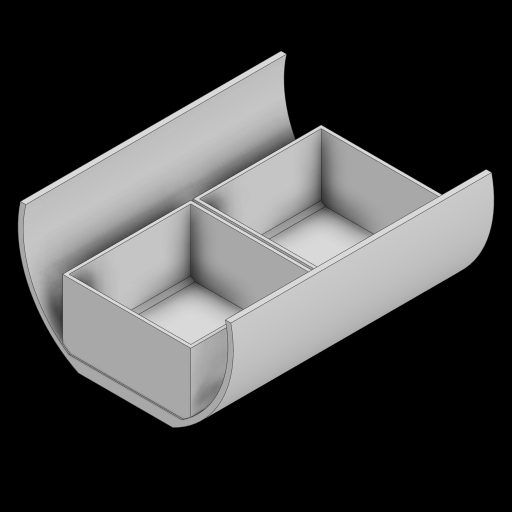
# Autodesk Inventor part: InsertV1
Saved by Autodesk Inventor 2024 (Build 280153000, 153)
## iProperties
Created: 2026-04-20
Part Number: InsertV1
Material: Generic
Document SubType Name: Modeling
Designer: Tanner
Density: 1 g/cm^3
Appearance: Default
Author: Tanner
## iProperties of the stored document InsertV1_3DPrint.ipt
Created: 2026-04-27
Part Number: InsertV1_3DPrint
Material: Generic
Document SubType Name: Modeling
Designer: Tanner
Density: 1 g/cm^3
Appearance: Default
Author: Tanner
Autodesk Inventor part; units mm, degrees
ref_plane "YZ Plane" through (0, 0, 0) normal (1, 0, 0) x (0, 1, 0)
ref_plane "XZ Plane" through (0, 0, 0) normal (0, 1, 0) x (-1, 0, 0)
ref_plane "XY Plane" through (0, 0, 0) normal (0, 0, 1) x (1, 0, 0)
sketch "Sketch1" plane through (0, 0, 0) normal (0, 0, 1) x (1, 0, 0)
  circle A0 centre (0, 0) radius 107.6 construction
  arc A1 (43.4971, -89.6) -> (-43.4971, -89.6) centre (0, 0) ccw construction
  line L0 (43.4971, -89.6) -> (-43.4971, -89.6) construction
  arc A2 (-96.8589, 20.9561) -> (-43.4971, -89.0439) centre (0, 0) ccw
  line L1 (-43.4971, -89.0439) -> (0, -89.0439)
  line L2 (-96.8589, 20.9561) -> (-91.8589, 20.9561)
  arc A3 (-91.8589, 20.9561) -> (-43.4971, -83.5776) centre (0, 0) ccw
  line L3 (-43.4971, -83.5776) -> (0, -83.5776)
  line L4 (0, 99.6) -> (0, -89.6) construction
  arc A4 (43.4971, -89.0439) -> (96.8589, 20.9561) centre (0, 0) ccw
  line L5 (43.4971, -89.0439) -> (0, -89.0439)
  line L6 (96.8589, 20.9561) -> (91.8589, 20.9561)
  arc A5 (43.4971, -83.5776) -> (91.8589, 20.9561) centre (0, 0) ccw
  line L7 (43.4971, -83.5776) -> (0, -83.5776)
  dimension "d0" = 0.5
  dimension "d1" = 110
  dimension "d2" = 5
  constraints: 14 end point, 9 point on circle, 4 centre point, 4 symmetric about line, 3 horizontal, 3 vertical alignment, 2 concentric, 1 midpoint, 2 other
  measures "d0" radial gap between concentric circles of A1 A2
  measures "d1" distance from line of L1 L2.start
  measures "d2" distance of L2.start L2.end
extrude "Extrusion1" add sketch "Sketch1" against normal blind 240
sketch "Sketch2" plane through (0, 0, 0) normal (0, 0, 1) x (1, 0, 0)
  line L0 (-50, -78.5776) -> (50, -78.5776) construction
  line L1 (50, -78.5776) -> (50, 21.4224) construction
  line L2 (-50, 21.4224) -> (50, 21.4224) construction
  line L3 (-50, -78.5776) -> (-50, 21.4224) construction
  arc A0 (-91.8589, 20.9561) -> (-43.4971, -83.5776) centre (0, 0) ccw projected
  line L4 (-51.9882, -78.5776) -> (51.9882, -78.5776)
  arc A1 (-51.9882, -78.5776) -> (-43.4971, -83.5776) centre (0, 0) ccw
  arc A2 (43.4971, -83.5776) -> (91.8589, 20.9561) centre (0, 0) ccw projected
  arc A3 (43.4971, -83.5776) -> (51.9882, -78.5776) centre (0, 0) ccw
  line L5 (43.4971, -83.5776) -> (-43.4971, -83.5776) projected
  line L6 (-43.4971, -83.5776) -> (43.4971, -83.5776)
  constraints: 5 point on circle, 4 end point, 2 centre point, 2 collinear, 2 concentric, 1 point on line
extrude "Extrusion2" add sketch "Sketch2" against normal up to surface (240 mm away)
sketch "Sketch3" plane through (-51.9882, -78.5776, 0) normal (0, 1, 0) x (1, 0, 0)
  line L0 (0, 240) -> (103.9765, 240) construction
  line L1 (0, 0) -> (0, 240) construction
  line L2 (103.9765, 0) -> (0, 0) construction
  line L3 (103.9765, 240) -> (103.9765, 0) construction
  line L4 (94.4882, 137.5) -> (9.4882, 137.5) construction
  line L5 (9.4882, 137.5) -> (9.4882, 222.5) construction
  line L6 (9.4882, 222.5) -> (94.4882, 222.5) construction
  line L7 (94.4882, 222.5) -> (94.4882, 137.5) construction
  line L8 (1.9882, 230) -> (1.9882, 130) construction
  line L9 (1.9882, 130) -> (101.9882, 130) construction
  line L10 (101.9882, 130) -> (101.9882, 230) construction
  line L11 (101.9882, 230) -> (1.9882, 230) construction
  line L12 (94.4882, 17.5) -> (9.4882, 17.5) construction
  line L13 (9.4882, 17.5) -> (9.4882, 102.5) construction
  line L14 (9.4882, 102.5) -> (94.4882, 102.5) construction
  line L15 (94.4882, 102.5) -> (94.4882, 17.5) construction
  line L16 (1.9882, 110) -> (1.9882, 10) construction
  line L17 (1.9882, 10) -> (101.9882, 10) construction
  line L18 (101.9882, 10) -> (101.9882, 110) construction
  line L19 (101.9882, 110) -> (1.9882, 110) construction
  line L20 (11.9882, 220) -> (11.9882, 140) construction
  line L21 (11.9882, 140) -> (91.9882, 140) construction
  line L22 (91.9882, 140) -> (91.9882, 220) construction
  line L23 (91.9882, 220) -> (11.9882, 220) construction
  line L24 (11.9882, 100) -> (11.9882, 20) construction
  line L25 (11.9882, 20) -> (91.9882, 20) construction
  line L26 (91.9882, 20) -> (91.9882, 100) construction
  line L27 (91.9882, 100) -> (11.9882, 100) construction
  line L28 (-4.0118, 124) -> (107.9882, 124)
  line L29 (107.9882, 124) -> (107.9882, 236)
  line L30 (107.9882, 236) -> (-4.0118, 236)
  line L31 (-4.0118, 236) -> (-4.0118, 124)
  line L32 (-4.0118, 124) -> (107.9882, 236) construction
  line L33 (107.9882, 124) -> (-4.0118, 236) construction
  line L34 (-7.0118, 121) -> (110.9882, 121)
  line L35 (110.9882, 121) -> (110.9882, 239)
  line L36 (110.9882, 239) -> (-7.0118, 239)
  line L37 (-7.0118, 239) -> (-7.0118, 121)
  line L38 (-7.0118, 121) -> (110.9882, 239) construction
  line L39 (110.9882, 121) -> (-7.0118, 239) construction
  line L40 (-4.0118, 4) -> (107.9882, 4)
  line L41 (107.9882, 4) -> (107.9882, 116)
  line L42 (107.9882, 116) -> (-4.0118, 116)
  line L43 (-4.0118, 116) -> (-4.0118, 4)
  line L44 (-4.0118, 4) -> (107.9882, 116) construction
  line L45 (107.9882, 4) -> (-4.0118, 116) construction
  line L46 (-7.0118, 1) -> (110.9882, 1)
  line L47 (110.9882, 1) -> (110.9882, 119)
  line L48 (110.9882, 119) -> (-7.0118, 119)
  line L49 (-7.0118, 119) -> (-7.0118, 1)
  line L50 (-7.0118, 1) -> (110.9882, 119) construction
  line L51 (110.9882, 1) -> (-7.0118, 119) construction
  point P0 (51.9882, 0)
  point P1 (51.9882, 180)
  point P2 (51.9882, 60)
  dimension "d7" = 6
  dimension "d8" = 6
  dimension "d9" = 6
  dimension "d10" = 6
  dimension "d11" = 3
  dimension "d12" = 6
  dimension "d13" = 6
  dimension "d14" = 6
  dimension "d15" = 6
  dimension "d16" = 3
  constraints: 48 end point, 8 midpoint, 8 parallel, 4 horizontal, 4 perpendicular, 2 point on line
  measures "d7" distance between parallel lines of L8 L31
  measures "d8" distance between parallel lines of L10 L29
  measures "d9" distance between parallel lines of L11 L30
  measures "d10" distance between parallel lines of L9 L28
  measures "d11" distance between parallel lines of L30 L36
  measures "d12" distance between parallel lines of L19 L42
  measures "d13" distance between parallel lines of L18 L41
  measures "d14" distance between parallel lines of L17 L40
  measures "d15" distance between parallel lines of L16 L43
  measures "d16" distance between parallel lines of L48 L42
extrude "Extrusion3" add sketch "Sketch3" along normal blind 60
body "Solid1"
